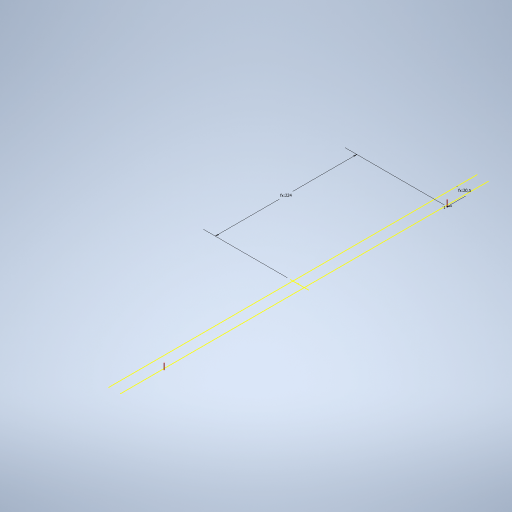
# Autodesk Inventor part: Shelf Holder Joint1200
Saved by Autodesk Inventor 2024 (Build 280153000, 153)
## iProperties
RuleStatus: InUse
Created: 2023-01-09
Part Number: Shelf Holder Joint1200
Material: Generic
Document SubType Name: Modeling
Designer: sauliusd
Density: 1 g/cm^3
Appearance: Default
AfterAnyUserParamChange0: ComponentsArrayParams
Author: sauliusd
Autodesk Inventor part; units mm, degrees
ref_plane "YZ Plane" through (0, 0, 0) normal (1, 0, 0) x (0, 1, 0)
ref_plane "XZ Plane" through (0, 0, 0) normal (0, 1, 0) x (-1, 0, 0)
ref_plane "XY Plane" through (0, 0, 0) normal (0, 0, 1) x (1, 0, 0)
sketch "Sketch1" plane through (0, 0, 0) normal (0, 0, 1) x (1, 0, 0)
  line L0 (-291.5, -9) -> (291.5, -9)
  line L1 (291.5, -9) -> (291.5, 9)
  line L2 (291.5, 9) -> (-291.5, 9)
  line L3 (-291.5, 9) -> (-291.5, -9)
  line L4 (-291.5, -9) -> (291.5, 9) construction
  line L5 (291.5, -9) -> (-291.5, 9) construction
  point P0 (0, 0)
  dimension "d0" = 583
  dimension "d1" = 18
  constraints: 12 end point, 2 midpoint, 2 parallel, 1 horizontal, 1 perpendicular
  measures "d0" distance of L2.end L1.end
  measures "d1" distance of L0.end L1.end
sketch "Lamello" plane through (0, 0, 0) normal (0, 0, 1) x (1, 0, 0)
  line L0 (48.383, 141.1858) -> (42.783, 141.1858)
  line L1 (40.583, 139.6858) -> (40.583, 114.6858)
  line L2 (42.783, 113.1858) -> (48.383, 113.1858)
  line L3 (50.583, 114.6858) -> (50.583, 139.6858)
  line L4 (50.583, 139.6858) -> (48.383, 141.1858)
  line L5 (40.583, 139.6858) -> (42.783, 141.1858)
  line L6 (40.583, 114.6858) -> (42.783, 113.1858)
  line L7 (50.583, 114.6858) -> (48.383, 113.1858)
  line L8 (50.583, 127.1858) -> (40.583, 127.1858)
  line L9 (45.583, 141.1858) -> (45.583, 113.1858)
  point P0 (45.583, 127.1858)
  point P1 (50.583, 141.1858)
  point P2 (40.583, 113.1858)
  point P3 (40.583, 141.1858)
  point P4 (50.583, 113.1858)
  dimension "d54" = 10
  dimension "d55" = 28
  dimension "d56" = 1.5
  dimension "d57" = 2.2
  dimension "d58" = 1.5
  dimension "d59" = 2.2
  dimension "d60" = 1.5
  dimension "d61" = 2.2
  dimension "d62" = 1.5
  dimension "d63" = 2.2
  measures "d54" distance of point (50.583, 113.186) point (40.583, 113.186)
  measures "d55" distance of point (40.583, 113.186) point (40.583, 141.186)
  measures "d56" distance of L3.end point (50.583, 141.186)
  measures "d57" distance of L0.start point (50.583, 141.186)
  measures "d58" distance of L1.start point (40.583, 141.186)
  measures "d59" distance of L0.end point (40.583, 141.186)
  measures "d60" distance of L1.end point (40.583, 113.186)
  measures "d61" distance of L2.start point (40.583, 113.186)
  measures "d62" distance of L3.start point (50.583, 113.186)
  measures "d63" distance of L2.end point (50.583, 113.186)
sketch "Sketch2" plane through (0, 0, 0) normal (0, 0, 1) x (1, 0, 0)
  circle A0 centre (224, -11.5) radius 0.5
  line L0 (291.5, 9) -> (-291.5, 9) projected
  line L1 (-291.5, -9) -> (291.5, -9) projected
  line L2 (0, -16.2) -> (0, 13.2) projected
  point P0 (0, 0)
  dimension "d2" = 224
  dimension "d4" = 1
  dimension "d50" = 20.5
  constraints: 1 centre point
  measures "d2" distance from line of A0.centre L2
  measures "d4" diameter of A0
  measures "d50" distance from line of L0 A0.centre
extrude "Extrusion1" add sketch "Sketch2" along normal blind 10
pattern_linear "Holders Array" count 2 spacing 448 along (-1, 0, 0) of "Extrusion1"
equation "\"d2\" = X_Coord"
equation "\"d9\" = Step"
equation "\"d0\" = ContactPatchWidth"
equation "\"d1\" = ContactPatchHeight"
equation "\"ContactPatchWidth\" = 583"
equation "\"ContactPatchHeight\" = 18"
equation "\"PlacingStep\" = 32"
equation "\"PlacingWidth\" = ContactPatchWidth - 2 * MinDistFromSide"
equation "\"MinDistBetween\" = 96"
equation "\"X_Coord\" = 224"
equation "\"Y_Coord\" = 0"
equation "\"NestleBoardT\" = 18"
equation "\"PillarBoardT\" = 18"
equation "\"AngleForYPositionCalc\" = 30deg"
equation "\"ConnectionAngle\" = 30deg"
equation "\"Step\" = 448"
equation "\"MinDistFromSide\" = 60"
